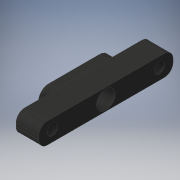
# Autodesk Inventor part: Fastener
Saved by Autodesk Inventor 2018 (Build 220112000, 112)
## iProperties
Created: 2018-10-18
Part Number: Fastener
Material: Generic
Document SubType Name: Modeling
Designer: USER
Density: 1 g/cm^3
Appearance: Rubber - Black
Author: USER
Autodesk Inventor part; units mm, degrees
ref_plane "YZ Plane" through (0, 0, 0) normal (1, 0, 0) x (0, 1, 0)
ref_plane "XZ Plane" through (0, 0, 0) normal (0, 1, 0) x (-1, 0, 0)
ref_plane "XY Plane" through (0, 0, 0) normal (0, 0, 1) x (1, 0, 0)
sketch "Sketch1" plane through (0, 0, 0) normal (1, 0, 0) x (0, 1, 0)
  line L0 (1.905, 0) -> (2.667, 0)
  line L1 (4.572, -1.905) -> (4.572, -27.559)
  line L2 (2.667, -29.464) -> (1.905, -29.464)
  line L3 (0, -27.559) -> (0, -1.905)
  arc A0 (4.572, -1.905) -> (2.667, 0) centre (2.667, -1.905) ccw
  arc A1 (1.905, 0) -> (0, -1.905) centre (1.905, -1.905) ccw
  arc A2 (0, -27.559) -> (1.905, -29.464) centre (1.905, -27.559) ccw
  arc A3 (2.667, -29.464) -> (4.572, -27.559) centre (2.667, -27.559) ccw
  circle A4 centre (2.286, -14.732) radius 1.5367
  point P0 (0, 0)
  point P1 (4.572, -29.464)
  point P2 (4.572, 0)
  point P3 (0, -29.464)
  dimension "d0" = 4.572
  dimension "d1" = 29.464
  dimension "d2" = 1.905
  dimension "d3" = 3.0734
  constraints: 8 end point, 8 point on circle, 8 point on line, 8 tangent, 5 centre point, 3 equal radius, 2 parallel, 1 coincident, 1 horizontal, 1 perpendicular
  measures "d0" distance of point (4.572, -29.464) point (0, -29.464)
  measures "d1" distance of point (4.572, 0) point (4.572, -29.464)
  measures "d2" radius of A0
  measures "d3" diameter of A4
extrude "Extrusion1" add sketch "Sketch1" along normal blind 5
sketch "Sketch2" plane through (0, 0, 0) normal (-1, 0, 0) x (0, 0, 1)
  circle A0 centre (-26.4658, 2.3835) radius 1.1682
  line L0 (-27.559, 4.572) -> (-1.905, 4.572) projected
  line L1 (-1.905, 0) -> (-27.559, 0) projected
  circle A1 centre (-2.9982, 2.3835) radius 1.1682
  point P0 (0, 0)
  constraints: 2 centre point
extrude "Extrusion2" cut sketch "Sketch2" against normal through all
sketch "Sketch3" plane through (0, 0, 0) normal (-1, 0, 0) x (0, 0, 1)
  line L0 (-20.3149, 2.2606) -> (-9.1747, 2.2606) construction
  line L1 (-20.3149, 4.5212) -> (-9.1747, 4.5212)
  line L2 (-9.1747, 0) -> (-20.3149, 0)
  arc A0 (-20.3149, 4.5212) -> (-20.3149, 0) centre (-20.3149, 2.2606) ccw
  arc A1 (-9.1747, 0) -> (-9.1747, 4.5212) centre (-9.1747, 2.2606) ccw
  point P0 (0, 0)
  point P1 (-14.7448, 2.2606)
  constraints: 8 end point, 4 point on circle, 4 tangent, 2 centre point, 1 horizontal, 1 midpoint, 1 parallel
extrude "Extrusion3" add sketch "Sketch3" along normal blind 2 separate body
sketch "Sketch4" plane through (-2, 0, 0) normal (-1, 0, 0) x (0, 0, 1)
  circle A0 centre (-14.7356, 2.2845) radius 1.5229
  point P0 (0, 0)
  constraints: 1 centre point
extrude "Extrusion4" cut sketch "Sketch4" against normal blind 2 bodies 2
sketch "Sketch5" plane through (-2, 0, 0) normal (-1, 0, 0) x (0, 0, 1)
  circle A0 centre (-14.7354, 2.2627) radius 2.0695
  point P0 (0, 0)
  constraints: 1 centre point
extrude "Extrusion5" cut sketch "Sketch5" against normal through all bodies 2
sketch "Sketch6" plane through (5, 0, 0) normal (1, 0, 0) x (0, 0, -1)
  circle A0 centre (14.7171, 2.2363) radius 2.0415
  point P0 (0, 0)
  constraints: 1 centre point
extrude "Extrusion6" cut sketch "Sketch6" against normal through all bodies 1
body "Solid1"
body "Solid2"
